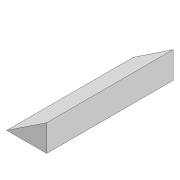
# Autodesk Inventor part: 200724 - 33-69 prism
Saved by Autodesk Inventor 2020.3 (Build 243373000, 373)
## iProperties
Created: 2020-07-24
Part Number: 200724 - 33-69 prism
Material: Generic
Document SubType Name: Modeling
Designer: Ralf
Density: 1 g/cm^3
Appearance: Default
Author: Ralf
Autodesk Inventor part; units mm, degrees
ref_plane "YZ Plane" through (0, 0, 0) normal (1, 0, 0) x (0, 1, 0)
ref_plane "XZ Plane" through (0, 0, 0) normal (0, 1, 0) x (-1, 0, 0)
ref_plane "XY Plane" through (0, 0, 0) normal (0, 0, 1) x (1, 0, 0)
sketch "Sketch1" plane through (0, 0, 0) normal (0, 0, 1) x (1, 0, 0)
  line L0 (0, 0) -> (6, 0)
  line L1 (0, 0) -> (6, 4)
  line L2 (0, 0) -> (7.2111, 0) construction
  line L3 (6, 4) -> (6, 0)
  dimension "d0" = 6
  dimension "d1" = 33.69
  constraints: 8 end point, 2 horizontal, 1 equal length, 1 vertical
  measures "d0" distance of L0.start L0.end
  measures "d1" angle of L2 L1
extrude "Extrusion1" add sketch "Sketch1" along normal blind 19
body "Solid1"
